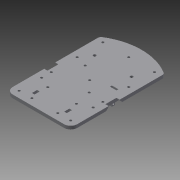
# Autodesk Inventor part: Bodenplatte_Motor2_liegend
Saved by Autodesk Inventor 2015 (Build 190159000, 159)
## iProperties
Created: 2015-03-02
Part Number: Bodenplatte_Motor2_liegend
Material: Generisch
Document SubType Name: Modeling
Designer: TowerSebi
Density: 1 g/cm^3
Appearance: Vorgabe
Author: TowerSebi
Autodesk Inventor part; units mm, degrees
ref_plane "YZ Plane" through (0, 0, 0) normal (1, 0, 0) x (0, 1, 0)
ref_plane "XZ Plane" through (0, 0, 0) normal (0, 1, 0) x (-1, 0, 0)
ref_plane "XY Plane" through (0, 0, 0) normal (0, 0, 1) x (1, 0, 0)
sketch "Skizze1" plane through (0, 0, 0) normal (0, 0, 1) x (1, 0, 0)
  line L0 (0, 0) -> (100, 0)
  line L1 (100, 0) -> (100, 145)
  line L2 (0, 145) -> (0, 0)
  arc A0 (100, 145) -> (0, 145) centre (50, 69.1667) ccw
  dimension "d0" = 145
  dimension "d1" = 100
  constraints: 6 end point, 2 point on circle, 1 centre point, 1 horizontal, 1 parallel, 1 perpendicular
  measures "d0" distance of L2.start L0.start
  measures "d1" distance of L1.end L2.start
extrude "Extrusion1" add sketch "Skizze1" along normal blind 5
fillet "Rundung2" radius 10 2 edges at (100, 0, 2.5) (0, 0, 2.5)
fillet "Rundung3" radius 5 2 edges at (100, 145, 2.5) (0, 145, 2.5)
sketch "Skizze3" plane through (0, 0, 0) normal (0, 0, -1) x (-1, 0, 0)
  line L0 (-10, 0) -> (-90, 0) projected
  line L1 (0, 142.2581) -> (0, 10) projected
  circle A0 centre (-90, 10) radius 1.75
  circle A1 centre (-70, 10) radius 1.75
  circle A2 centre (-30, 10) radius 1.75
  circle A3 centre (-10, 10) radius 1.75
  circle A4 centre (-10, 60) radius 1.75
  circle A5 centre (-10, 100) radius 1.75
  circle A6 centre (-10, 140) radius 1.75
  circle A7 centre (-50, 140) radius 1.75
  circle A8 centre (-90, 140) radius 1.75
  circle A9 centre (-90, 100) radius 1.75
  circle A10 centre (-90, 60) radius 1.75
  point P0 (0, 0)
  dimension "d12" = 3.5
  dimension "d13" = 3.5
  dimension "d14" = 3.5
  dimension "d15" = 3.5
  dimension "d16" = 3.5
  dimension "d17" = 3.5
  dimension "d18" = 3.5
  dimension "d19" = 3.5
  dimension "d20" = 3.5
  dimension "d21" = 3.5
  dimension "d22" = 3.5
  dimension "d23" = 140
  dimension "d24" = 140
  dimension "d25" = 140
  dimension "d26" = 100
  dimension "d27" = 100
  dimension "d28" = 60
  dimension "d29" = 60
  dimension "d30" = 10
  dimension "d31" = 10
  dimension "d32" = 10
  dimension "d33" = 10
  dimension "d34" = 90
  dimension "d35" = 70
  dimension "d36" = 30
  dimension "d37" = 10
  dimension "d38" = 90
  dimension "d39" = 10
  dimension "d40" = 90
  dimension "d41" = 10
  dimension "d42" = 90
  dimension "d43" = 50
  dimension "d44" = 10
  constraints: 11 centre point
  measures "d12" diameter of A8
  measures "d13" diameter of A7
  measures "d14" diameter of A6
  measures "d15" diameter of A9
  measures "d16" diameter of A5
  measures "d17" diameter of A10
  measures "d18" diameter of A4
  measures "d19" diameter of A0
  measures "d20" diameter of A1
  measures "d21" diameter of A2
  measures "d22" diameter of A3
  measures "d23" distance from line of L0 A8.centre
  measures "d24" distance from line of L0 A7.centre
  measures "d25" distance from line of L0 A6.centre
  measures "d26" distance from line of L0 A9.centre
  measures "d27" distance from line of L0 A5.centre
  measures "d28" distance from line of L0 A10.centre
  measures "d29" distance from line of L0 A4.centre
  measures "d30" distance from line of L0 A0.centre
  measures "d31" distance from line of A1.centre L0
  measures "d32" distance from line of L0 A2.centre
  measures "d33" distance from line of L0 A3.centre
  measures "d34" distance from line of L1 A0.centre
  measures "d35" distance from line of L1 A1.centre
  measures "d36" distance from line of A2.centre L1
  measures "d37" distance of L1.end A3.centre
  measures "d38" distance from line of L1 A10.centre
  measures "d39" distance from line of L1 A4.centre
  measures "d40" distance from line of L1 A9.centre
  measures "d41" distance from line of L1 A5.centre
  measures "d42" distance from line of A8.centre L1
  measures "d43" distance from line of L1 A7.centre
  measures "d44" distance from line of L1 A6.centre
extrude "Extrusion2" cut sketch "Skizze3" against normal up to next
sketch "Skizze4" plane through (0, 0, 0) normal (0, 0, -1) x (-1, 0, 0)
  circle A0 centre (-90, 100) radius 1.75 projected
  circle A1 centre (-50, 140) radius 1.75 projected
  circle A2 centre (-10, 100) radius 1.75 projected
  circle A3 centre (-10, 10) radius 1.75 projected
  circle A4 centre (-70, 10) radius 1.75 projected
  circle A5 centre (-90, 10) radius 1.75 projected
  circle A6 centre (-30, 10) radius 1.75 projected
  circle A7 centre (-10, 60) radius 1.75 projected
  circle A8 centre (-10, 140) radius 1.75 projected
  circle A9 centre (-90, 140) radius 1.75 projected
  circle A10 centre (-90, 60) radius 1.75 projected
  arc A11 (-100, 10) -> (-90, 0) centre (-90, 10) ccw projected
  arc A12 (-10, 0) -> (0, 10) centre (-10, 10) ccw projected
  line L0 (-87.1442, 138.3646) -> (-89.9884, 136.7091)
  line L1 (-89.9884, 136.7091) -> (-92.8442, 138.3445)
  line L2 (-92.8442, 138.3445) -> (-92.8558, 141.6354)
  line L3 (-92.8558, 141.6354) -> (-90.0116, 143.2909)
  line L4 (-90.0116, 143.2909) -> (-87.1558, 141.6555)
  line L5 (-87.1558, 141.6555) -> (-87.1442, 138.3646)
  line L6 (-47.1806, 138.3027) -> (-50.0602, 136.7097)
  line L7 (-50.0602, 136.7097) -> (-52.8796, 138.407)
  line L8 (-52.8796, 138.407) -> (-52.8194, 141.6973)
  line L9 (-52.8194, 141.6973) -> (-49.9398, 143.2903)
  line L10 (-49.9398, 143.2903) -> (-47.1204, 141.593)
  line L11 (-47.1204, 141.593) -> (-47.1806, 138.3027)
  line L12 (-87.1903, 98.2866) -> (-90.079, 96.7101)
  line L13 (-90.079, 96.7101) -> (-92.8887, 98.4234)
  line L14 (-92.8887, 98.4234) -> (-92.8097, 101.7134)
  line L15 (-92.8097, 101.7134) -> (-89.921, 103.2899)
  line L16 (-89.921, 103.2899) -> (-87.1113, 101.5766)
  line L17 (-87.1113, 101.5766) -> (-87.1903, 98.2866)
  line L18 (-92.8311, 58.3222) -> (-92.8686, 61.6129)
  line L19 (-92.8686, 61.6129) -> (-90.0375, 63.2907)
  line L20 (-90.0375, 63.2907) -> (-87.1689, 61.6778)
  line L21 (-87.1689, 61.6778) -> (-87.1314, 58.3871)
  line L22 (-87.1314, 58.3871) -> (-89.9625, 56.7093)
  line L23 (-89.9625, 56.7093) -> (-92.8311, 58.3222)
  line L24 (-92.8568, 8.3664) -> (-92.8431, 11.6573)
  line L25 (-92.8431, 11.6573) -> (-89.9863, 13.2909)
  line L26 (-89.9863, 13.2909) -> (-87.1432, 11.6336)
  line L27 (-87.1432, 11.6336) -> (-87.1569, 8.3427)
  line L28 (-87.1569, 8.3427) -> (-90.0137, 6.7091)
  line L29 (-90.0137, 6.7091) -> (-92.8568, 8.3664)
  line L30 (-72.859, 8.3702) -> (-72.8409, 11.6611)
  line L31 (-72.8409, 11.6611) -> (-69.9819, 13.2908)
  line L32 (-69.9819, 13.2908) -> (-67.141, 11.6298)
  line L33 (-67.141, 11.6298) -> (-67.1591, 8.3389)
  line L34 (-67.1591, 8.3389) -> (-70.0181, 6.7092)
  line L35 (-70.0181, 6.7092) -> (-72.859, 8.3702)
  line L36 (-30, 6.7091) -> (-32.85, 8.3546)
  line L37 (-32.85, 8.3546) -> (-32.85, 11.6454)
  line L38 (-32.85, 11.6454) -> (-30, 13.2909)
  line L39 (-30, 13.2909) -> (-27.15, 11.6454)
  line L40 (-27.15, 11.6454) -> (-27.15, 8.3546)
  line L41 (-27.15, 8.3546) -> (-30, 6.7091)
  line L42 (-10, 6.7091) -> (-12.85, 8.3546)
  line L43 (-12.85, 8.3546) -> (-12.85, 11.6454)
  line L44 (-12.85, 11.6454) -> (-10, 13.2909)
  line L45 (-10, 13.2909) -> (-7.15, 11.6454)
  line L46 (-7.15, 11.6454) -> (-7.15, 8.3546)
  line L47 (-7.15, 8.3546) -> (-10, 6.7091)
  line L48 (-10, 56.7091) -> (-12.85, 58.3546)
  line L49 (-12.85, 58.3546) -> (-12.85, 61.6454)
  line L50 (-12.85, 61.6454) -> (-10, 63.2909)
  line L51 (-10, 63.2909) -> (-7.15, 61.6454)
  line L52 (-7.15, 61.6454) -> (-7.15, 58.3546)
  line L53 (-7.15, 58.3546) -> (-10, 56.7091)
  line L54 (-10, 96.7091) -> (-12.85, 98.3546)
  line L55 (-12.85, 98.3546) -> (-12.85, 101.6454)
  line L56 (-12.85, 101.6454) -> (-10, 103.2909)
  line L57 (-10, 103.2909) -> (-7.15, 101.6454)
  line L58 (-7.15, 101.6454) -> (-7.15, 98.3546)
  line L59 (-7.15, 98.3546) -> (-10, 96.7091)
  line L60 (-10, 136.7091) -> (-12.85, 138.3546)
  line L61 (-12.85, 138.3546) -> (-12.85, 141.6454)
  line L62 (-12.85, 141.6454) -> (-10, 143.2909)
  line L63 (-10, 143.2909) -> (-7.15, 141.6454)
  line L64 (-7.15, 141.6454) -> (-7.15, 138.3546)
  line L65 (-7.15, 138.3546) -> (-10, 136.7091)
  point P0 (0, 0)
  dimension "d49" = 5.7
  dimension "d50" = 5.7
  dimension "d51" = 5.7
  dimension "d52" = 5.7
  dimension "d53" = 5.7
  dimension "d54" = 5.7
  dimension "d55" = 5.7
  dimension "d56" = 5.7
  dimension "d57" = 5.7
  dimension "d58" = 5.7
  dimension "d59" = 5.7
  constraints: 132 end point, 11 coincident, 143 other
  measures "d49" distance between parallel lines of L0 L3
  measures "d50" distance between parallel lines of L13 L16
  measures "d51" distance between parallel lines of L23 L20
  measures "d52" distance between parallel lines of L28 L25
  measures "d53" distance between parallel lines of L34 L31
  measures "d54" distance between parallel lines of L41 L38
  measures "d55" distance between parallel lines of L47 L44
  measures "d56" distance between parallel lines of L53 L50
  measures "d57" distance between parallel lines of L59 L56
  measures "d58" distance between parallel lines of L65 L62
  measures "d59" distance between parallel lines of L10 L7
extrude "Extrusion3" cut sketch "Skizze4" against normal blind 4.3
sketch "Skizze5" plane through (0, 0, 0) normal (0, 0, -1) x (-1, 0, 0)
  line L0 (-100, 10) -> (-100, 142.2581) projected
  line L1 (-10, 0) -> (-90, 0) projected
  line L2 (0, 142.2581) -> (0, 10) projected
  circle A0 centre (-78.5, 116) radius 2.15
  circle A1 centre (-21.25, 116) radius 2.15
  point P0 (0, 0)
  dimension "d62" = 4.3
  dimension "d63" = 4.3
  dimension "d64" = 116
  dimension "d65" = 116
  dimension "d66" = 21.5
  dimension "d67" = 57.25
  dimension "d68" = 21.25
  constraints: 2 centre point
  measures "d62" diameter of A0
  measures "d63" diameter of A1
  measures "d64" distance from line of A1.centre L1
  measures "d65" distance from line of L1 A0.centre
  measures "d66" distance from line of L0 A0.centre
  measures "d67" distance of A1.centre A0.centre
  measures "d68" distance from line of L2 A1.centre
extrude "Extrusion4" cut sketch "Skizze5" against normal up to next
sketch "Skizze6" plane through (0, 0, 0) normal (0, 0, -1) x (-1, 0, 0)
  line L0 (-10, 0) -> (-90, 0) projected
  line L1 (0, 142.2581) -> (0, 10) projected
  circle A0 centre (-50, 152.5) radius 5
  point P0 (0, 0)
  dimension "d71" = 10
  dimension "d72" = 50
  dimension "d73" = 152.5
  constraints: 1 centre point
  measures "d71" diameter of A0
  measures "d72" distance from line of L1 A0.centre
  measures "d73" distance from line of L0 A0.centre
extrude "Extrusion5" add sketch "Skizze6" along normal blind 22
fillet "Rundung4" radius 5 1 edges at (55, 152.5, -22)
sketch "Skizze7" plane through (0, 0, 0) normal (0, 0, -1) x (-1, 0, 0)
  line L0 (-100, 10) -> (-100, 142.2581) projected
  line L1 (-10, 0) -> (-90, 0) projected
  line L2 (0, 142.2581) -> (0, 10) projected
  line L3 (-84.4, 84.5) -> (-79.4, 84.5)
  line L4 (-79.4, 84.5) -> (-79.4, 79.5)
  line L5 (-79.4, 79.5) -> (-84.4, 79.5)
  line L6 (-84.4, 79.5) -> (-84.4, 84.5)
  line L7 (-20.6, 84.5) -> (-15.6, 84.5)
  line L8 (-15.6, 84.5) -> (-15.6, 79.5)
  line L9 (-15.6, 79.5) -> (-20.6, 79.5)
  line L10 (-20.6, 79.5) -> (-20.6, 84.5)
  line L11 (-77, 52.5) -> (-72, 52.5)
  line L12 (-72, 52.5) -> (-72, 42.5)
  line L13 (-72, 42.5) -> (-77, 42.5)
  line L14 (-77, 42.5) -> (-77, 52.5)
  line L15 (-28, 52.5) -> (-23, 52.5)
  line L16 (-23, 52.5) -> (-23, 42.5)
  line L17 (-23, 42.5) -> (-28, 42.5)
  line L18 (-28, 42.5) -> (-28, 52.5)
  point P0 (0, 0)
  dimension "d77" = 5
  dimension "d78" = 5
  dimension "d79" = 5
  dimension "d80" = 5
  dimension "d81" = 5
  dimension "d82" = 5
  dimension "d83" = 10
  dimension "d84" = 10
  dimension "d85" = 42.5
  dimension "d86" = 42.5
  dimension "d87" = 79.5
  dimension "d88" = 79.5
  dimension "d89" = 23
  dimension "d90" = 23
  dimension "d91" = 15.6
  dimension "d92" = 15.6
  constraints: 32 end point, 8 parallel, 4 horizontal, 4 perpendicular
  measures "d77" distance of L11.start L11.end
  measures "d78" distance between parallel lines of L18 L16
  measures "d79" distance of L8.end L9.end
  measures "d80" distance of L4.end L5.end
  measures "d81" distance of L7.end L8.end
  measures "d82" distance of L3.end L4.end
  measures "d83" distance of L13.end L11.start
  measures "d84" distance of L15.end L16.end
  measures "d85" distance between parallel lines of L1 L13
  measures "d86" distance between parallel lines of L1 L17
  measures "d87" distance between parallel lines of L1 L9
  measures "d88" distance between parallel lines of L1 L5
  measures "d89" distance between parallel lines of L0 L14
  measures "d90" distance between parallel lines of L2 L16
  measures "d91" distance between parallel lines of L0 L6
  measures "d92" distance between parallel lines of L2 L8
extrude "Extrusion6" add sketch "Skizze7" along normal blind 23
sketch "Skizze8" plane through (77, 42.5, 0) normal (1, 0, 0) x (0, 0, -1)
  line L0 (23, 10) -> (23, 0) projected
  line L1 (0, 10) -> (23, 10) projected
  circle A0 centre (3, 5) radius 1.75
  circle A1 centre (20.5, 5) radius 1.75
  point P0 (0, -42.5)
  dimension "d95" = 2.5
  dimension "d97" = 20
  dimension "d98" = 3.5
  dimension "d99" = 3.5
  dimension "d100" = 5
  constraints: 2 centre point
  measures "d95" distance from line of L0 A1.centre
  measures "d97" distance from line of L0 A0.centre
  measures "d98" diameter of A0
  measures "d99" diameter of A1
  measures "d100" distance from line of L1 A1.centre
extrude "Extrusion7" cut sketch "Skizze8" against normal through all
hole "Bohrung1" at (84.4, 82, -11.5) direction (-1, 0, 0) diameter 3 end through all
sketch "Skizze9" plane through (84.4, 79.5, 0) normal (1, 0, 0) x (0, 0, -1)
  line L0 (23, 5) -> (23, 0) projected
  line L1 (0, 5) -> (23, 5) projected
  line L2 (0, 0) -> (23, 0) projected
  line L3 (14, 5) -> (14, 0)
  circle A0 centre (11.5, 2.5) radius 1.5 projected
  point P0 (0, -79.5)
  dimension "d116" = 2.5
  constraints: 2 end point, 2 point on line, 1 perpendicular
  measures "d116" distance from line of A0.centre L3
extrude "Extrusion8" cut sketch "Skizze9" against normal through all contours L0 L2 L3 L1
sketch "Skizze10" plane through (0, 0, 5) normal (0, 0, 1) x (1, 0, 0)
  line L0 (10, 0) -> (90, 0) projected
  line L1 (100, 10) -> (100, 142.2581) projected
  circle A0 centre (10, 45) radius 1.75
  circle A1 centre (90, 45) radius 1.75
  point P0 (0, 0)
  dimension "d124" = 3.5
  dimension "d125" = 3.5
  dimension "d126" = 10
  dimension "d127" = 90
  dimension "d128" = 45
  dimension "d129" = 45
  constraints: 2 centre point
  measures "d124" diameter of A0
  measures "d125" diameter of A1
  measures "d126" distance from line of L1 A1.centre
  measures "d127" distance from line of L1 A0.centre
  measures "d128" distance from line of A0.centre L0
  measures "d129" distance from line of L0 A1.centre
extrude "Extrusion9" cut sketch "Skizze10" against normal up to next
sketch "Skizze11" plane through (0, 0, 0) normal (0, 0, -1) x (-1, 0, 0)
  circle A0 centre (-10, 45) radius 1.75 projected
  circle A1 centre (-90, 45) radius 1.75 projected
  line L0 (-90, 48.2909) -> (-87.15, 46.6454)
  line L1 (-87.15, 46.6454) -> (-87.15, 43.3546)
  line L2 (-87.15, 43.3546) -> (-90, 41.7091)
  line L3 (-90, 41.7091) -> (-92.85, 43.3546)
  line L4 (-92.85, 43.3546) -> (-92.85, 46.6454)
  line L5 (-92.85, 46.6454) -> (-90, 48.2909)
  line L6 (-10, 48.2909) -> (-7.15, 46.6454)
  line L7 (-7.15, 46.6454) -> (-7.15, 43.3546)
  line L8 (-7.15, 43.3546) -> (-10, 41.7091)
  line L9 (-10, 41.7091) -> (-12.85, 43.3546)
  line L10 (-12.85, 43.3546) -> (-12.85, 46.6454)
  line L11 (-12.85, 46.6454) -> (-10, 48.2909)
  point P0 (0, 0)
  dimension "d132" = 5.7
  dimension "d133" = 5.7
  constraints: 24 end point, 2 coincident, 26 other
  measures "d132" distance between parallel lines of L5 L2
  measures "d133" distance between parallel lines of L11 L8
extrude "Extrusion10" cut sketch "Skizze11" against normal blind 4.3
sketch "Skizze12" plane through (0, 0, 0) normal (0, 0, -1) x (-1, 0, 0)
  line L0 (-100, 10) -> (-100, 142.2581) projected
  line L1 (-10, 0) -> (-90, 0) projected
  line L2 (0, 142.2581) -> (0, 10) projected
  line L3 (-85, 89) -> (-75, 89)
  line L4 (-75, 89) -> (-75, 86)
  line L5 (-75, 86) -> (-85, 86)
  line L6 (-85, 86) -> (-85, 89)
  line L7 (-77, 25) -> (-73, 25)
  line L8 (-73, 25) -> (-73, 17)
  line L9 (-73, 17) -> (-77, 17)
  line L10 (-77, 17) -> (-77, 25)
  line L11 (-23, 17) -> (-27, 17)
  line L12 (-27, 17) -> (-27, 25)
  line L13 (-27, 25) -> (-23, 25)
  line L14 (-23, 25) -> (-23, 17)
  point P0 (0, 0)
  dimension "d136" = 4
  dimension "d137" = 4
  dimension "d138" = 3
  dimension "d139" = 10
  dimension "d140" = 8
  dimension "d141" = 8
  dimension "d142" = 17
  dimension "d143" = 17
  dimension "d144" = 23
  dimension "d145" = 23
  dimension "d146" = 15
  dimension "d147" = 86
  constraints: 24 end point, 6 parallel, 3 horizontal, 3 perpendicular
  measures "d136" distance of L7.start L7.end
  measures "d137" distance of L12.end L13.end
  measures "d138" distance of L3.end L4.end
  measures "d139" distance of L4.end L5.end
  measures "d140" distance between parallel lines of L7 L9
  measures "d141" distance of L11.end L12.end
  measures "d142" distance between parallel lines of L1 L9
  measures "d143" distance between parallel lines of L1 L11
  measures "d144" distance between parallel lines of L14 L2
  measures "d145" distance between parallel lines of L0 L10
  measures "d146" distance between parallel lines of L0 L6
  measures "d147" distance between parallel lines of L1 L5
extrude "Extrusion11" cut sketch "Skizze12" against normal up to next
sketch "Skizze13" plane through (0, 0, 5) normal (0, 0, 1) x (1, 0, 0)
  line L0 (0, 142.2581) -> (0, 10) projected
  line L1 (10, 0) -> (90, 0) projected
  circle A0 centre (27.5, 37) radius 1.75
  circle A1 centre (72, 37) radius 1.75
  circle A2 centre (50.5, 79) radius 1.75
  circle A3 centre (27.5, 95) radius 1.75
  circle A4 centre (66.8, 62) radius 1.75
  point P0 (0, 0)
  dimension "d150" = 3.5
  dimension "d151" = 3.5
  dimension "d152" = 3.5
  dimension "d156" = 27.5
  dimension "d157" = 37
  dimension "d158" = 37
  dimension "d159" = 3.5
  dimension "d160" = 3.5
  dimension "d162" = 27.5
  dimension "d174" = 44.5
  dimension "d175" = 42
  dimension "d177" = 23
  dimension "d178" = 95
  dimension "d179" = 39.3
  dimension "d180" = 33
  constraints: 5 centre point
  measures "d150" diameter of A2
  measures "d151" diameter of A1
  measures "d152" diameter of A0
  measures "d156" distance from line of L0 A0.centre
  measures "d157" distance from line of L1 A0.centre
  measures "d158" distance from line of L1 A1.centre
  measures "d159" diameter of A3
  measures "d160" diameter of A4
  measures "d162" distance from line of L0 A3.centre
  measures "d174" distance of A1.centre A0.centre
  measures "d175" vertical distance of A2.centre A0.centre
  measures "d177" horizontal distance of A2.centre A0.centre
  measures "d178" distance from line of A3.centre L1
  measures "d179" horizontal distance of A3.centre A4.centre
  measures "d180" vertical distance of A4.centre A3.centre
extrude "Extrusion12" cut sketch "Skizze13" against normal up to next
sketch "Skizze14" plane through (0, 0, 0) normal (0, 0, -1) x (-1, 0, 0)
  circle A0 centre (-27.5, 95) radius 1.75 projected
  circle A1 centre (-72, 37) radius 1.75 projected
  circle A2 centre (-27.5, 37) radius 1.75 projected
  circle A3 centre (-50.5, 79) radius 1.75 projected
  circle A4 centre (-66.8, 62) radius 1.75 projected
  line L0 (-50.5, 82.2909) -> (-47.65, 80.6454)
  line L1 (-47.65, 80.6454) -> (-47.65, 77.3546)
  line L2 (-47.65, 77.3546) -> (-50.5, 75.7091)
  line L3 (-50.5, 75.7091) -> (-53.35, 77.3546)
  line L4 (-53.35, 77.3546) -> (-53.35, 80.6454)
  line L5 (-53.35, 80.6454) -> (-50.5, 82.2909)
  line L6 (-27.5, 98.2909) -> (-24.65, 96.6454)
  line L7 (-24.65, 96.6454) -> (-24.65, 93.3546)
  line L8 (-24.65, 93.3546) -> (-27.5, 91.7091)
  line L9 (-27.5, 91.7091) -> (-30.35, 93.3546)
  line L10 (-30.35, 93.3546) -> (-30.35, 96.6454)
  line L11 (-30.35, 96.6454) -> (-27.5, 98.2909)
  line L12 (-27.5, 40.2909) -> (-24.65, 38.6454)
  line L13 (-24.65, 38.6454) -> (-24.65, 35.3546)
  line L14 (-24.65, 35.3546) -> (-27.5, 33.7091)
  line L15 (-27.5, 33.7091) -> (-30.35, 35.3546)
  line L16 (-30.35, 35.3546) -> (-30.35, 38.6454)
  line L17 (-30.35, 38.6454) -> (-27.5, 40.2909)
  line L18 (-66.8, 65.2909) -> (-63.95, 63.6454)
  line L19 (-63.95, 63.6454) -> (-63.95, 60.3546)
  line L20 (-63.95, 60.3546) -> (-66.8, 58.7091)
  line L21 (-66.8, 58.7091) -> (-69.65, 60.3546)
  line L22 (-69.65, 60.3546) -> (-69.65, 63.6454)
  line L23 (-69.65, 63.6454) -> (-66.8, 65.2909)
  line L24 (-72.0118, 40.2909) -> (-69.1559, 38.6557)
  line L25 (-69.1559, 38.6557) -> (-69.1441, 35.3648)
  line L26 (-69.1441, 35.3648) -> (-71.9882, 33.7091)
  line L27 (-71.9882, 33.7091) -> (-74.8441, 35.3443)
  line L28 (-74.8441, 35.3443) -> (-74.8559, 38.6352)
  line L29 (-74.8559, 38.6352) -> (-72.0118, 40.2909)
  point P0 (0, 0)
  dimension "d167" = 5.7
  dimension "d168" = 5.7
  dimension "d169" = 5.7
  dimension "d170" = 5.7
  dimension "d171" = 5.7
  constraints: 60 end point, 5 coincident, 65 other
  measures "d167" distance between parallel lines of L26 L29
  measures "d168" distance between parallel lines of L20 L23
  measures "d169" distance between parallel lines of L14 L17
  measures "d170" distance between parallel lines of L11 L8
  measures "d171" distance between parallel lines of L5 L2
extrude "Extrusion13" cut sketch "Skizze14" against normal blind 4.3
fillet "Rundung7" radius 3 1 edges at (55, 152.5, 0)
sketch "Skizze15" plane through (0, 0, 5) normal (0, 0, 1) x (1, 0, 0)
  line L0 (0, 142.2581) -> (0, 10) projected
  line L1 (10, 0) -> (90, 0) projected
  line L2 (100, 10) -> (100, 142.2581) projected
  line L3 (0, 76) -> (5, 76)
  line L4 (5, 76) -> (5, 59)
  line L5 (5, 59) -> (0, 59)
  line L6 (0, 59) -> (0, 76)
  line L7 (100, 76) -> (95, 76)
  line L8 (95, 76) -> (95, 59)
  line L9 (95, 59) -> (100, 59)
  line L10 (100, 59) -> (100, 76)
  point P0 (0, 0)
  dimension "d183" = 59
  dimension "d184" = 59
  dimension "d185" = 17
  dimension "d186" = 17
  dimension "d187" = 5
  dimension "d188" = 5
  constraints: 16 end point, 4 parallel, 2 horizontal, 2 perpendicular, 2 point on line
  measures "d183" distance between parallel lines of L1 L5
  measures "d184" distance between parallel lines of L1 L9
  measures "d185" distance between parallel lines of L9 L7
  measures "d186" distance between parallel lines of L5 L3
  measures "d187" distance of L3.start L3.end
  measures "d188" distance of L7.start L7.end
extrude "Extrusion14" cut sketch "Skizze15" against normal up to next
chamfer "Fase1" distance 4 angle 45 4 edges at (97.5, 76, 0) (97.5, 59, 0) (2.5, 76, 0) (2.5, 59, 0)
